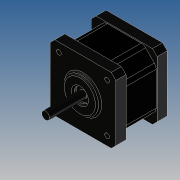
# Autodesk Inventor part: 3211_Stepper Motor_V1
Saved by Autodesk Inventor 2020 (Build 240168000, 168)
## iProperties
Created: 2019-11-01
Part Number: 3211_Stepper Motor_V1
Material: Stainless Steel, Brushed
Document SubType Name: Modeling
Designer: RFLab
Density: 8 g/cm^3
Appearance: Stainless - Brushed
Mass: 623.493 g
Surface Area: 119.127 cm^2
Volume: 77.9366 cm^3
Author: RFLab
Autodesk Inventor part; units mm, degrees
ref_plane "YZ Plane" through (0, 0, 0) normal (1, 0, 0) x (0, 1, 0)
ref_plane "XZ Plane" through (0, 0, 0) normal (0, 1, 0) x (-1, 0, 0)
ref_plane "XY Plane" through (0, 0, 0) normal (0, 0, 1) x (1, 0, 0)
sketch "Sketch1" plane through (0, 0, 0) normal (0, 0, 1) x (1, 0, 0)
  line L0 (-18.15, -21.15) -> (18.15, -21.15)
  line L1 (21.15, -18.15) -> (21.15, 18.15)
  line L2 (18.15, 21.15) -> (-18.15, 21.15)
  line L3 (-21.15, 18.15) -> (-21.15, -18.15)
  line L4 (-21.15, -21.15) -> (21.15, 21.15) construction
  line L5 (21.15, -21.15) -> (-21.15, 21.15) construction
  line L6 (-21.15, 18.15) -> (-18.15, 21.15)
  line L7 (18.15, 21.15) -> (21.15, 18.15)
  line L8 (21.15, -18.15) -> (18.15, -21.15)
  line L9 (-18.15, -21.15) -> (-21.15, -18.15)
  line L10 (-15.5, -15.5) -> (15.5, -15.5) construction
  line L11 (15.5, -15.5) -> (15.5, 15.5) construction
  line L12 (15.5, 15.5) -> (-15.5, 15.5) construction
  line L13 (-15.5, 15.5) -> (-15.5, -15.5) construction
  line L14 (-15.5, -15.5) -> (15.5, 15.5) construction
  line L15 (15.5, -15.5) -> (-15.5, 15.5) construction
  circle A0 centre (-15.5, 15.5) radius 1.5
  circle A1 centre (15.5, 15.5) radius 1.5
  circle A2 centre (15.5, -15.5) radius 1.5
  circle A3 centre (-15.5, -15.5) radius 1.5
  point P0 (0, 0)
  dimension "d0" = 42.3
  dimension "d1" = 42.3
  dimension "d2" = 3
  dimension "d3" = 3
  dimension "d4" = 3
  dimension "d5" = 3
  dimension "d6" = 3
  dimension "d7" = 3
  dimension "d8" = 3
  dimension "d9" = 3
  dimension "d10" = 31
  dimension "d11" = 31
  dimension "d12" = 3
  dimension "d13" = 3
  dimension "d14" = 3
  dimension "d15" = 3
  constraints: 32 end point, 8 point on line, 4 centre point, 4 coincident, 4 midpoint, 4 parallel, 2 horizontal, 2 perpendicular
  measures "d0" distance of L5.end L4.end
  measures "d1" distance of L4.end L5.start
  measures "d2" distance of L3.start L5.end
  measures "d3" distance of L2.end L5.end
  measures "d4" distance of L2.start L4.end
  measures "d5" distance of L1.end L4.end
  measures "d6" distance of L1.start L5.start
  measures "d7" distance of L0.end L5.start
  measures "d8" distance of L0.start L4.start
  measures "d9" distance of L3.end L4.start
  measures "d10" distance of L12.end L11.end
  measures "d11" distance of L11.end L10.end
  measures "d12" diameter of A0
  measures "d13" diameter of A2
  measures "d14" diameter of A3
  measures "d15" diameter of A1
extrude "Extrusion1" add sketch "Sketch1" along normal mid plane 33
sketch "Sketch2" plane through (0, 0, 0) normal (0, 0, 1) x (1, 0, 0)
  circle A0 centre (-15.5, 15.5) radius 1.5 projected
  circle A1 centre (15.5, 15.5) radius 1.5 projected
  circle A2 centre (15.5, -15.5) radius 1.5 projected
  circle A3 centre (-15.5, -15.5) radius 1.5 projected
  point P0 (0, 0)
extrude "Extrusion2" add sketch "Sketch2" along normal mid plane 20
sketch "Sketch3" plane through (0, 0, 0) normal (0, 0, 1) x (1, 0, 0)
  line L0 (10.8431, -20.5) -> (-10.8431, -20.5)
  line L1 (-20.5, -10.8431) -> (-20.5, 10.8431)
  line L2 (-10.8431, 20.5) -> (10.8431, 20.5)
  line L3 (20.5, 10.8431) -> (20.5, -10.8431)
  line L4 (20.5, -20.5) -> (-20.5, 20.5) construction
  line L5 (-20.5, -20.5) -> (20.5, 20.5) construction
  line L6 (-19.3284, 13.6716) -> (-13.6716, 19.3284)
  line L7 (13.6716, 19.3284) -> (19.3284, 13.6716)
  line L8 (19.3284, -13.6716) -> (13.6716, -19.3284)
  line L9 (-13.6716, -19.3284) -> (-19.3284, -13.6716)
  arc A0 (-10.8431, 20.5) -> (-13.6716, 19.3284) centre (-10.8431, 16.5) ccw
  arc A1 (-19.3284, 13.6716) -> (-20.5, 10.8431) centre (-16.5, 10.8431) ccw
  arc A2 (13.6716, 19.3284) -> (10.8431, 20.5) centre (10.8431, 16.5) ccw
  arc A3 (20.5, 10.8431) -> (19.3284, 13.6716) centre (16.5, 10.8431) ccw
  arc A4 (19.3284, -13.6716) -> (20.5, -10.8431) centre (16.5, -10.8431) ccw
  arc A5 (10.8431, -20.5) -> (13.6716, -19.3284) centre (10.8431, -16.5) ccw
  arc A6 (-13.6716, -19.3284) -> (-10.8431, -20.5) centre (-10.8431, -16.5) ccw
  arc A7 (-20.5, -10.8431) -> (-19.3284, -13.6716) centre (-16.5, -10.8431) ccw
  line L10 (-21.15, 18.15) -> (-18.15, 21.15) projected
  line L11 (-18.15, 21.15) -> (18.15, 21.15) projected
  line L12 (18.15, 21.15) -> (21.15, 18.15) projected
  line L13 (21.15, 18.15) -> (21.15, -18.15) projected
  line L14 (21.15, -18.15) -> (18.15, -21.15) projected
  line L15 (18.15, -21.15) -> (-18.15, -21.15) projected
  line L16 (-18.15, -21.15) -> (-21.15, -18.15) projected
  line L17 (-21.15, -18.15) -> (-21.15, 18.15) projected
  circle A8 centre (-15.5, 15.5) radius 1.5 projected
  circle A9 centre (15.5, 15.5) radius 1.5 projected
  circle A10 centre (15.5, -15.5) radius 1.5 projected
  circle A11 centre (-15.5, -15.5) radius 1.5 projected
  point P0 (0, 0)
  point P1 (-20.5, 12.5)
  point P2 (-12.5, 20.5)
  point P3 (12.5, 20.5)
  point P4 (20.5, 12.5)
  point P5 (20.5, -12.5)
  point P6 (12.5, -20.5)
  point P7 (-12.5, -20.5)
  point P8 (-20.5, -12.5)
  point P9 (-11.3431, -21.15)
  point P10 (-21.15, -11.4931)
  point P11 (11.3431, -21.15)
  point P12 (21.15, -11.4931)
  point P13 (21.15, 11.4931)
  point P14 (11.3431, 21.15)
  point P15 (-11.3431, 21.15)
  point P16 (-21.15, 11.4931)
  dimension "d20" = 41
  dimension "d21" = 41
  dimension "d22" = 8
  dimension "d23" = 8
  dimension "d24" = 8
  dimension "d25" = 8
  dimension "d26" = 8
  dimension "d27" = 8
  dimension "d28" = 8
  dimension "d29" = 8
  dimension "d30" = 4
  constraints: 24 point on line, 20 end point, 16 point on circle, 16 tangent, 8 centre point, 7 equal radius, 2 midpoint, 2 parallel, 1 horizontal, 1 perpendicular
  measures "d20" distance of L4.end L5.end
  measures "d21" distance of L5.start L4.end
  measures "d22" distance of point (-20.5, 12.5) L4.end
  measures "d23" distance of point (-12.5, 20.5) L4.end
  measures "d24" distance of point (12.5, 20.5) L5.end
  measures "d25" distance of point (20.5, 12.5) L5.end
  measures "d26" distance of point (20.5, -12.5) L4.start
  measures "d27" distance of point (12.5, -20.5) L4.start
  measures "d28" distance of point (-12.5, -20.5) L5.start
  measures "d29" distance of point (-20.5, -12.5) L5.start
  measures "d30" radius of A0
extrude "Extrusion3" cut sketch "Sketch3" along normal mid plane 20 contours L8 A10 | A11 L9 | L7 A9 | A8 L6 | L10 L11 L12 L13 L14 L15 L16 L17 picked at (16.5579, -16.478) picked at (-16.478, -16.5579) picked at (16.5579, 16.478) picked at (-16.5579, 16.478)
sketch "Sketch4" plane through (0, 0, 16.5) normal (0, 0, 1) x (1, 0, 0)
  circle A0 centre (0, 0) radius 11
  dimension "d33" = 22
  constraints: 1 centre point, 1 coincident
  measures "d33" diameter of A0
extrude "Extrusion4" add sketch "Sketch4" along normal blind 2
sketch "Sketch5" plane through (0, 0, 18.5) normal (0, 0, 1) x (1, 0, 0)
  circle A0 centre (0, 0) radius 2.5
  dimension "d36" = 5
  constraints: 1 centre point, 1 coincident
  measures "d36" diameter of A0
extrude "Extrusion5" add sketch "Sketch5" along normal blind 22
sketch "Sketch6" plane through (0, 0, 18.5) normal (0, 0, 1) x (1, 0, 0)
  circle A0 centre (0, 0) radius 2.5 projected
  circle A1 centre (0, 0) radius 4.5
  dimension "d39" = 2
  constraints: 1 centre point
  measures "d39" radial gap between concentric circles of A0 A1
extrude "Extrusion6" cut sketch "Sketch6" against normal blind 2
fillet "Fillet1" radius 1 3 edges at (-11, 0, 16.5) (-4.5, 0, 18.5) (-11, 0, 18.5)
equation "\"d3\" = d2"
equation "\"d4\" = d2"
equation "\"d5\" = d4"
equation "\"d6\" = d2"
equation "\"d7\" = d6"
equation "\"d8\" = d2"
equation "\"d9\" = d8"
equation "\"d23\" = d22"
equation "\"d24\" = d22"
equation "\"d25\" = d24"
equation "\"d26\" = d22"
equation "\"d27\" = d26"
equation "\"d28\" = d22"
equation "\"d29\" = d28"
body "Solid1"
